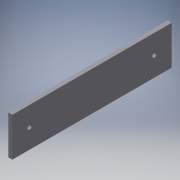
# Autodesk Inventor part: Mechanum support lock bar
Saved by Autodesk Inventor 2018 (Build 220112000, 112)
## iProperties
Created: 2018-05-02
Part Number: Mechanum support lock bar
Material: Generic
Document SubType Name: Modeling
Designer: Ajith Thomas
Density: 1 g/cm^3
Appearance: Default
Author: Ajith Thomas
Autodesk Inventor part; units mm, degrees
ref_plane "YZ Plane" through (0, 0, 0) normal (1, 0, 0) x (0, 1, 0)
ref_plane "XZ Plane" through (0, 0, 0) normal (0, 1, 0) x (-1, 0, 0)
ref_plane "XY Plane" through (0, 0, 0) normal (0, 0, 1) x (1, 0, 0)
sketch "Sketch1" plane through (0, 0, 0) normal (0, 0, 1) x (1, 0, 0)
  line L0 (-25.1745, 14) -> (-25.1745, -14) projected
  line L1 (-25.1745, 14) -> (-22.1745, 14)
  line L2 (-22.1745, 14) -> (-22.1745, -14)
  line L3 (-22.1745, -14) -> (-25.1745, -14)
  line L4 (-25.1745, -14) -> (-25.1745, 14)
  point P0 (0, 0)
  dimension "d0" = 3
  dimension "d1" = 28
  constraints: 8 end point, 2 parallel, 1 horizontal, 1 perpendicular
  measures "d0" distance of L2.end L3.end
  measures "d1" distance between parallel lines of L3 L1
extrude "Extrusion1" add sketch "Sketch1" along normal mid plane 115
sketch "Sketch2" plane through (-25.1745, -14, 57.5) normal (-1, 0, 0) x (0, 0, 1)
  line L0 (-115, 0) -> (-115, 28) construction
  line L1 (0, 28) -> (0, 0) construction
  line L2 (0, 0) -> (-115, 0) construction
  line L3 (-115, 28) -> (0, 28) construction
  line L4 (-57.5, 0) -> (-57.5, 28) construction
  circle A0 centre (-12.5, 14) radius 1.5
  circle A1 centre (-102.5, 14) radius 1.5
  point P0 (-57.5, 14)
  dimension "d4" = 3
  dimension "d5" = 12.5
  dimension "d6" = 14
  constraints: 2 centre point, 2 end point, 2 midpoint, 1 symmetric about line, 1 other
  measures "d4" diameter of A0
  measures "d5" distance from line of L1 A0.centre
  measures "d6" distance from line of L2 A0.centre
extrude "Extrusion2" cut sketch "Sketch2" against normal blind 10
body "Solid1"
